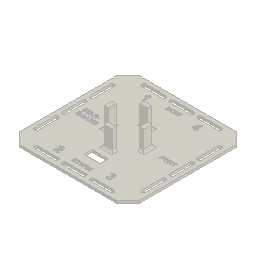
Top Plate (Autodesk Fusion 360 design; units mm, degrees)
Autodesk Fusion 360 part; units mm, degrees
sketch "Sketch1" plane through (0, 0, 0) normal (0, 0, 1) x (1, 0, 0)
  line L0 (0, 0) -> (150, 0)
  line L1 (150, 0) -> (150, 150)
  line L2 (150, 150) -> (0, 150)
  line L3 (0, 150) -> (0, 0)
  line L4 (0, 135.8579) -> (14.1421, 150)
  line L5 (0, 135.8579) -> (21.2132, 135.8579) construction
  line L6 (150, 135.8579) -> (135.8579, 150)
  line L7 (150, 135.8579) -> (176.9741, 135.8579) construction
  line L8 (0, 14.1421) -> (14.1421, 0)
  line L9 (0, 14.1421) -> (24.9877, 14.1421) construction
  line L10 (135.8579, 0) -> (150, 14.1421)
  line L11 (135.8579, 0) -> (156.2132, 0) construction
  line L12 (75, 150) -> (75, 0) construction
  line L13 (0, 75) -> (150, 75) construction
  line L14 (65, 40) -> (85, 40)
  line L15 (85, 40) -> (85, 30)
  line L16 (85, 30) -> (65, 30)
  line L17 (65, 30) -> (65, 40)
  line L18 (62, 145) -> (88, 145)
  line L19 (90, 143) -> (90, 142)
  line L20 (88, 140) -> (62, 140)
  line L21 (60, 142) -> (60, 143)
  line L22 (97, 145) -> (123, 145)
  line L23 (125, 143) -> (125, 142)
  line L24 (123, 140) -> (97, 140)
  line L25 (95, 142) -> (95, 143)
  line L26 (53, 145) -> (27, 145)
  line L27 (25, 143) -> (25, 142)
  line L28 (27, 140) -> (53, 140)
  line L29 (55, 142) -> (55, 143)
  arc A0 (27, 145) -> (25, 143) centre (27, 143) ccw
  arc A1 (25, 142) -> (27, 140) centre (27, 142) ccw
  arc A2 (53, 140) -> (55, 142) centre (53, 142) ccw
  arc A3 (55, 143) -> (53, 145) centre (53, 143) ccw
  arc A4 (62, 145) -> (60, 143) centre (62, 143) ccw
  arc A5 (60, 142) -> (62, 140) centre (62, 142) ccw
  arc A6 (90, 143) -> (88, 145) centre (88, 143) ccw
  arc A7 (88, 140) -> (90, 142) centre (88, 142) ccw
  arc A8 (95, 142) -> (97, 140) centre (97, 142) ccw
  arc A9 (97, 145) -> (95, 143) centre (97, 143) ccw
  arc A10 (125, 143) -> (123, 145) centre (123, 143) ccw
  arc A11 (123, 140) -> (125, 142) centre (123, 142) ccw
  line L30 (5, 53) -> (5, 27)
  line L31 (5, 97) -> (5, 123)
  arc A12 (10, 88) -> (8, 90) centre (8, 88) ccw
  arc A13 (8, 60) -> (10, 62) centre (8, 62) ccw
  line L32 (10, 88) -> (10, 62)
  line L33 (7, 25) -> (8, 25)
  line L34 (10, 123) -> (10, 97)
  line L35 (10, 27) -> (10, 53)
  line L36 (8, 60) -> (7, 60)
  line L37 (5, 62) -> (5, 88)
  arc A14 (7, 55) -> (5, 53) centre (7, 53) ccw
  arc A15 (10, 53) -> (8, 55) centre (8, 53) ccw
  arc A16 (5, 27) -> (7, 25) centre (7, 27) ccw
  arc A17 (7, 90) -> (5, 88) centre (7, 88) ccw
  arc A18 (8, 95) -> (10, 97) centre (8, 97) ccw
  arc A19 (10, 123) -> (8, 125) centre (8, 123) ccw
  arc A20 (7, 125) -> (5, 123) centre (7, 123) ccw
  line L38 (8, 55) -> (7, 55)
  arc A21 (5, 97) -> (7, 95) centre (7, 97) ccw
  arc A22 (5, 62) -> (7, 60) centre (7, 62) ccw
  line L39 (7, 90) -> (8, 90)
  line L40 (8, 95) -> (7, 95)
  line L41 (7, 125) -> (8, 125)
  arc A23 (8, 25) -> (10, 27) centre (8, 27) ccw
  line L42 (97, 5) -> (123, 5)
  line L43 (53, 5) -> (27, 5)
  arc A24 (62, 10) -> (60, 8) centre (62, 8) ccw
  arc A25 (90, 8) -> (88, 10) centre (88, 8) ccw
  line L44 (62, 10) -> (88, 10)
  line L45 (125, 7) -> (125, 8)
  line L46 (27, 10) -> (53, 10)
  line L47 (123, 10) -> (97, 10)
  line L48 (90, 8) -> (90, 7)
  line L49 (88, 5) -> (62, 5)
  arc A26 (95, 7) -> (97, 5) centre (97, 7) ccw
  arc A27 (97, 10) -> (95, 8) centre (97, 8) ccw
  arc A28 (123, 5) -> (125, 7) centre (123, 7) ccw
  arc A29 (60, 7) -> (62, 5) centre (62, 7) ccw
  arc A30 (55, 8) -> (53, 10) centre (53, 8) ccw
  arc A31 (27, 10) -> (25, 8) centre (27, 8) ccw
  arc A32 (25, 7) -> (27, 5) centre (27, 7) ccw
  line L50 (95, 8) -> (95, 7)
  arc A33 (53, 5) -> (55, 7) centre (53, 7) ccw
  arc A34 (88, 5) -> (90, 7) centre (88, 7) ccw
  line L51 (60, 7) -> (60, 8)
  line L52 (55, 8) -> (55, 7)
  line L53 (25, 7) -> (25, 8)
  arc A35 (125, 8) -> (123, 10) centre (123, 8) ccw
  line L54 (145, 97) -> (145, 123)
  line L55 (145, 53) -> (145, 27)
  arc A36 (140, 62) -> (142, 60) centre (142, 62) ccw
  arc A37 (142, 90) -> (140, 88) centre (142, 88) ccw
  line L56 (140, 62) -> (140, 88)
  line L57 (143, 125) -> (142, 125)
  line L58 (140, 27) -> (140, 53)
  line L59 (140, 123) -> (140, 97)
  line L60 (142, 90) -> (143, 90)
  line L61 (145, 88) -> (145, 62)
  arc A38 (143, 95) -> (145, 97) centre (143, 97) ccw
  arc A39 (140, 97) -> (142, 95) centre (142, 97) ccw
  arc A40 (145, 123) -> (143, 125) centre (143, 123) ccw
  arc A41 (143, 60) -> (145, 62) centre (143, 62) ccw
  arc A42 (142, 55) -> (140, 53) centre (142, 53) ccw
  arc A43 (140, 27) -> (142, 25) centre (142, 27) ccw
  arc A44 (143, 25) -> (145, 27) centre (143, 27) ccw
  line L62 (142, 95) -> (143, 95)
  arc A45 (145, 53) -> (143, 55) centre (143, 53) ccw
  arc A46 (145, 88) -> (143, 90) centre (143, 88) ccw
  line L63 (143, 60) -> (142, 60)
  line L64 (142, 55) -> (143, 55)
  line L65 (143, 25) -> (142, 25)
  arc A47 (142, 125) -> (140, 123) centre (142, 123) ccw
  point P0 (60, 145)
  point P1 (90, 145)
  point P2 (125, 145)
  point P3 (125, 140)
  point P4 (75, 75)
  point P5 (5, 125)
  point P6 (5, 90)
  point P7 (10, 125)
  point P8 (5, 60)
  point P9 (25, 5)
  point P10 (60, 5)
  point P11 (25, 10)
  point P12 (90, 5)
  point P13 (145, 25)
  point P14 (145, 60)
  point P15 (140, 25)
  point P16 (145, 90)
  point P17 (75, 145)
  dimension "d5" = 150
  dimension "d6" = 150
  dimension "d7" = 45
  dimension "d8" = 135
  dimension "d9" = 45
  dimension "d10" = 45
  dimension "d11" = 20
  dimension "d14" = 20
  dimension "d15" = 10
  dimension "d16" = 10
  dimension "d17" = 30
  dimension "d18" = 30
  dimension "d21" = 5
  dimension "d22" = 5
  dimension "d23" = 2
  dimension "d24" = 5
  dimension "d25" = 5
  dimension "d27" = 360
  constraint horizontal L0
  constraint vertical L1
  constraint horizontal L2
  constraint vertical L3
  constraint coincident L0.start L3.end
  constraint horizontal L5
  constraint coincident L3 L4.start
  constraint coincident L2 L4.end
  constraint horizontal L7
  constraint coincident L1 L6.start
  constraint coincident L2 L6.end
  constraint horizontal L9
  constraint coincident L3 L8.start
  constraint coincident L0 L8.end
  constraint horizontal L11
  constraint coincident L0 L10.start
  constraint coincident L1 L10.end
  constraint equal L4 L6
  constraint equal L6 L10
  constraint equal L8 L10
  constraint midpoint L2 L12.start
  constraint midpoint L0 L12.end
  constraint midpoint L3 L13.start
  constraint midpoint L1 L13.end
  constraint horizontal L14
  constraint vertical L15
  constraint horizontal L16
  constraint vertical L17
  constraint horizontal L18
  constraint vertical L19
  constraint horizontal L20
  constraint vertical L21
  constraint horizontal L22
  constraint vertical L23
  constraint horizontal L24
  constraint vertical L25
  constraint horizontal L26
  constraint vertical L27
  constraint horizontal L28
  constraint vertical L29
  constraint collinear L18 L26
  constraint collinear L18 L22
  constraint collinear L20 L28
  constraint collinear L20 L24
  constraint tangent L26 A0
  constraint tangent L27 A0
  constraint tangent L27 A1
  constraint tangent L28 A1
  constraint equal A0 A1
  constraint tangent L28 A2
  constraint tangent L29 A2
  constraint equal A0 A2
  constraint tangent L26 A3
  constraint tangent L29 A3
  constraint equal A0 A3
  constraint coincident P0 L18
  constraint coincident P0 L21
  constraint tangent L18 A4
  constraint tangent L21 A4
  constraint equal A0 A4
  constraint tangent L20 A5
  constraint tangent L21 A5
  constraint equal A0 A5
  constraint coincident P1 L18
  constraint coincident P1 L19
  constraint tangent L18 A6
  constraint tangent L19 A6
  constraint equal A0 A6
  constraint tangent L19 A7
  constraint tangent L20 A7
  constraint equal A0 A7
  constraint tangent L24 A8
  constraint tangent L25 A8
  constraint equal A0 A8
  constraint tangent L22 A9
  constraint tangent L25 A9
  constraint equal A0 A9
  constraint coincident P2 L22
  constraint coincident P2 L23
  constraint tangent L22 A10
  constraint tangent L23 A10
  constraint equal A0 A10
  constraint coincident P3 L23
  constraint coincident P3 L24
  constraint tangent L23 A11
  constraint tangent L24 A11
  constraint equal A0 A11
  constraint midpoint L13 P4
  constraint midpoint L18 P17
  constraint coincident L12 P17
  constraint equal L18 L22
  constraint equal L18 L26
  measures "d5" distance of L0.start L0.end
  measures "d6" distance of L0.start L2.end
  measures "d7" angle of L4 L5
  measures "d8" angle of L6 L7
  measures "d9" angle of L8 L9
  measures "d10" angle of L10 L11
  measures "d11" distance of L10.start L10.end
  measures "d14" distance of L15.end L16.end
  measures "d15" distance of L12 L17
  measures "d16" distance of L14.start L16.end
  measures "d17" distance of L0 L16
  measures "d18" distance of P0 P1
  measures "d21" distance of L2 L22
  measures "d22" distance of P2 P3
  measures "d23" radius of A0
  measures "d24" distance of L21 L29
  measures "d25" distance of L19 L25
extrude "Extrude1" add sketch "Sketch1" along normal blind 3 contours L0 L1 L2 L3 L4 L6 L8 L10
sketch "Sketch2" plane through (0, 0, 3) normal (0, 0, 1) x (-1, 0, 0)
  arc A0 (-5, -62) -> (-7, -60) centre (-7, -62) ccw
  line L0 (-5, -62) -> (-5, -88)
  arc A1 (-7, -90) -> (-5, -88) centre (-7, -88) ccw
  line L1 (-7, -90) -> (-8, -90)
  arc A2 (-10, -88) -> (-8, -90) centre (-8, -88) ccw
  line L2 (-10, -88) -> (-10, -62)
  arc A3 (-8, -60) -> (-10, -62) centre (-8, -62) ccw
  line L3 (-8, -60) -> (-7, -60)
  arc A4 (-142, -125) -> (-140, -123) centre (-142, -123) ccw
  line L4 (-142, -125) -> (-143, -125)
  arc A5 (-145, -123) -> (-143, -125) centre (-143, -123) ccw
  line L5 (-145, -123) -> (-145, -97)
  arc A6 (-143, -95) -> (-145, -97) centre (-143, -97) ccw
  line L6 (-143, -95) -> (-142, -95)
  arc A7 (-140, -97) -> (-142, -95) centre (-142, -97) ccw
  line L7 (-140, -97) -> (-140, -123)
  arc A8 (-88, -5) -> (-90, -7) centre (-88, -7) ccw
  line L8 (-88, -5) -> (-62, -5)
  arc A9 (-60, -7) -> (-62, -5) centre (-62, -7) ccw
  line L9 (-60, -7) -> (-60, -8)
  arc A10 (-62, -10) -> (-60, -8) centre (-62, -8) ccw
  line L10 (-62, -10) -> (-88, -10)
  arc A11 (-90, -8) -> (-88, -10) centre (-88, -8) ccw
  line L11 (-90, -8) -> (-90, -7)
  arc A12 (-145, -53) -> (-143, -55) centre (-143, -53) ccw
  line L12 (-145, -53) -> (-145, -27)
  arc A13 (-143, -25) -> (-145, -27) centre (-143, -27) ccw
  line L13 (-143, -25) -> (-142, -25)
  arc A14 (-140, -27) -> (-142, -25) centre (-142, -27) ccw
  line L14 (-140, -27) -> (-140, -53)
  arc A15 (-142, -55) -> (-140, -53) centre (-142, -53) ccw
  line L15 (-142, -55) -> (-143, -55)
  arc A16 (-125, -8) -> (-123, -10) centre (-123, -8) ccw
  line L16 (-125, -8) -> (-125, -7)
  arc A17 (-123, -5) -> (-125, -7) centre (-123, -7) ccw
  line L17 (-123, -5) -> (-97, -5)
  arc A18 (-95, -7) -> (-97, -5) centre (-97, -7) ccw
  line L18 (-95, -7) -> (-95, -8)
  arc A19 (-97, -10) -> (-95, -8) centre (-97, -8) ccw
  line L19 (-97, -10) -> (-123, -10)
  arc A20 (-53, -5) -> (-55, -7) centre (-53, -7) ccw
  line L20 (-53, -5) -> (-27, -5)
  arc A21 (-25, -7) -> (-27, -5) centre (-27, -7) ccw
  line L21 (-25, -7) -> (-25, -8)
  arc A22 (-27, -10) -> (-25, -8) centre (-27, -8) ccw
  line L22 (-27, -10) -> (-53, -10)
  arc A23 (-55, -8) -> (-53, -10) centre (-53, -8) ccw
  line L23 (-55, -8) -> (-55, -7)
  arc A24 (-145, -88) -> (-143, -90) centre (-143, -88) ccw
  line L24 (-145, -88) -> (-145, -62)
  arc A25 (-143, -60) -> (-145, -62) centre (-143, -62) ccw
  line L25 (-143, -60) -> (-142, -60)
  arc A26 (-140, -62) -> (-142, -60) centre (-142, -62) ccw
  line L26 (-140, -62) -> (-140, -88)
  arc A27 (-142, -90) -> (-140, -88) centre (-142, -88) ccw
  line L27 (-142, -90) -> (-143, -90)
  arc A28 (-5, -97) -> (-7, -95) centre (-7, -97) ccw
  line L28 (-5, -97) -> (-5, -123)
  arc A29 (-7, -125) -> (-5, -123) centre (-7, -123) ccw
  line L29 (-7, -125) -> (-8, -125)
  arc A30 (-10, -123) -> (-8, -125) centre (-8, -123) ccw
  line L30 (-10, -123) -> (-10, -97)
  arc A31 (-8, -95) -> (-10, -97) centre (-8, -97) ccw
  line L31 (-8, -95) -> (-7, -95)
  arc A32 (-95, -142) -> (-97, -140) centre (-97, -142) ccw
  line L32 (-95, -142) -> (-95, -143)
  arc A33 (-97, -145) -> (-95, -143) centre (-97, -143) ccw
  line L33 (-97, -145) -> (-123, -145)
  arc A34 (-125, -143) -> (-123, -145) centre (-123, -143) ccw
  line L34 (-125, -143) -> (-125, -142)
  arc A35 (-123, -140) -> (-125, -142) centre (-123, -142) ccw
  line L35 (-123, -140) -> (-97, -140)
  arc A36 (-60, -142) -> (-62, -140) centre (-62, -142) ccw
  line L36 (-60, -142) -> (-60, -143)
  arc A37 (-62, -145) -> (-60, -143) centre (-62, -143) ccw
  line L37 (-62, -145) -> (-88, -145)
  arc A38 (-90, -143) -> (-88, -145) centre (-88, -143) ccw
  line L38 (-90, -143) -> (-90, -142)
  arc A39 (-88, -140) -> (-90, -142) centre (-88, -142) ccw
  line L39 (-88, -140) -> (-62, -140)
  arc A40 (-55, -143) -> (-53, -145) centre (-53, -143) ccw
  line L40 (-55, -143) -> (-55, -142)
  arc A41 (-53, -140) -> (-55, -142) centre (-53, -142) ccw
  line L41 (-53, -140) -> (-27, -140)
  arc A42 (-25, -142) -> (-27, -140) centre (-27, -142) ccw
  line L42 (-25, -142) -> (-25, -143)
  arc A43 (-27, -145) -> (-25, -143) centre (-27, -143) ccw
  line L43 (-27, -145) -> (-53, -145)
  arc A44 (-8, -25) -> (-10, -27) centre (-8, -27) ccw
  line L44 (-8, -25) -> (-7, -25)
  arc A45 (-5, -27) -> (-7, -25) centre (-7, -27) ccw
  line L45 (-5, -27) -> (-5, -53)
  arc A46 (-7, -55) -> (-5, -53) centre (-7, -53) ccw
  line L46 (-7, -55) -> (-8, -55)
  arc A47 (-10, -53) -> (-8, -55) centre (-8, -53) ccw
  line L47 (-10, -53) -> (-10, -27)
  line L48 (-85, -30) -> (-65, -30)
  line L49 (-65, -30) -> (-65, -40)
  line L50 (-65, -40) -> (-85, -40)
  line L51 (-85, -40) -> (-85, -30)
  line L52 (0, -135.8579) -> (0, -14.1421)
  line L53 (0, -14.1421) -> (-14.1421, 0)
  line L54 (-14.1421, 0) -> (-135.8579, 0)
  line L55 (-135.8579, 0) -> (-150, -14.1421)
  line L56 (-150, -14.1421) -> (-150, -135.8579)
  line L57 (-150, -135.8579) -> (-135.8579, -150)
  line L58 (-135.8579, -150) -> (-14.1421, -150)
  line L59 (-14.1421, -150) -> (0, -135.8579)
  line L60 (0, 0) -> (-150, 0) construction
  line L61 (-150, 0) -> (-150, -150) construction
  line L62 (-150, -150) -> (0, -150) construction
  line L63 (0, -150) -> (0, 0) construction
  line L64 (0, -75) -> (-150, -75) construction
  line L65 (-75, -150) -> (-75, 0) construction
  line L66 (-70, -100) -> (-80, -100)
  line L67 (-80, -100) -> (-80, -95)
  line L68 (-80, -95) -> (-70, -95)
  line L69 (-70, -95) -> (-70, -100)
  line L70 (-55, -70) -> (-50, -70)
  line L71 (-55, -80) -> (-55, -70)
  line L72 (-50, -70) -> (-50, -80)
  line L73 (-50, -80) -> (-55, -80)
  line L74 (-80, -55) -> (-80, -50)
  line L75 (-70, -55) -> (-80, -55)
  line L76 (-80, -50) -> (-70, -50)
  line L77 (-70, -50) -> (-70, -55)
  line L78 (-95, -80) -> (-100, -80)
  line L79 (-95, -70) -> (-95, -80)
  line L80 (-100, -80) -> (-100, -70)
  line L81 (-100, -70) -> (-95, -70)
  point P0 (-75, -75)
  dimension "d28" = 10
  dimension "d29" = 5
  dimension "d30" = 5
  dimension "d31" = 20
  dimension "d33" = 360
  constraint horizontal L60
  constraint vertical L61
  constraint horizontal L62
  constraint vertical L63
  constraint coincident L60.start L63.end
  constraint midpoint L63 L64.start
  constraint midpoint L61 L64.end
  constraint midpoint L62 L65.start
  constraint midpoint L60 L65.end
  constraint horizontal L66
  constraint vertical L67
  constraint horizontal L68
  constraint vertical L69
  constraint midpoint L65 P0
  measures "d28" distance of L66.start L66.end
  measures "d29" distance of L65 L69
  measures "d30" distance of L66.end L67.end
  measures "d31" distance of L64 L68
extrude "Extrude2" add sketch "Sketch2" along normal blind 25 contours L66 L67 L68 L69 | L70 L71 L72 L73 | L74 L75 L76 L77 | L78 L79 L80 L81
fillet "Fillet1" radius 3 12 edges at (75, 50, 3) (80, 52.5, 3) (97.5, 70, 3) (100, 75, 3) (52.5, 70, 3) (70, 52.5, 3) (50, 75, 3) (70, 97.5, 3) (97.5, 80, 3) (75, 100, 3) (52.5, 80, 3) (80, 97.5, 3)
sketch "Sketch3" plane through (0, 0, 3) normal (0, 0, 1) x (-1, 0, 0)
  line L0 (-67, -55) -> (-83, -55)
  line L1 (-83, -55) -> (-83, -47)
  line L2 (-83, -47) -> (-67, -47)
  line L3 (-67, -47) -> (-67, -55)
  line L4 (-83, -95) -> (-67, -95)
  line L5 (-67, -95) -> (-67, -103)
  line L6 (-67, -103) -> (-83, -103)
  line L7 (-83, -103) -> (-83, -95)
  line L8 (-95, -67) -> (-95, -83)
  line L9 (-95, -83) -> (-103, -83)
  line L10 (-103, -83) -> (-103, -67)
  line L11 (-103, -67) -> (-95, -67)
  arc A0 (-5, -62) -> (-7, -60) centre (-7, -62) ccw
  line L12 (-5, -62) -> (-5, -88)
  arc A1 (-7, -90) -> (-5, -88) centre (-7, -88) ccw
  line L13 (-7, -90) -> (-8, -90)
  arc A2 (-10, -88) -> (-8, -90) centre (-8, -88) ccw
  line L14 (-10, -88) -> (-10, -62)
  arc A3 (-8, -60) -> (-10, -62) centre (-8, -62) ccw
  line L15 (-8, -60) -> (-7, -60)
  arc A4 (-142, -125) -> (-140, -123) centre (-142, -123) ccw
  line L16 (-142, -125) -> (-143, -125)
  arc A5 (-145, -123) -> (-143, -125) centre (-143, -123) ccw
  line L17 (-145, -123) -> (-145, -97)
  arc A6 (-143, -95) -> (-145, -97) centre (-143, -97) ccw
  line L18 (-143, -95) -> (-142, -95)
  arc A7 (-140, -97) -> (-142, -95) centre (-142, -97) ccw
  line L19 (-140, -97) -> (-140, -123)
  arc A8 (-88, -5) -> (-90, -7) centre (-88, -7) ccw
  line L20 (-88, -5) -> (-62, -5)
  arc A9 (-60, -7) -> (-62, -5) centre (-62, -7) ccw
  line L21 (-60, -7) -> (-60, -8)
  arc A10 (-62, -10) -> (-60, -8) centre (-62, -8) ccw
  line L22 (-62, -10) -> (-88, -10)
  arc A11 (-90, -8) -> (-88, -10) centre (-88, -8) ccw
  line L23 (-90, -8) -> (-90, -7)
  arc A12 (-145, -53) -> (-143, -55) centre (-143, -53) ccw
  line L24 (-145, -53) -> (-145, -27)
  arc A13 (-143, -25) -> (-145, -27) centre (-143, -27) ccw
  line L25 (-143, -25) -> (-142, -25)
  arc A14 (-140, -27) -> (-142, -25) centre (-142, -27) ccw
  line L26 (-140, -27) -> (-140, -53)
  arc A15 (-142, -55) -> (-140, -53) centre (-142, -53) ccw
  line L27 (-142, -55) -> (-143, -55)
  arc A16 (-125, -8) -> (-123, -10) centre (-123, -8) ccw
  line L28 (-125, -8) -> (-125, -7)
  arc A17 (-123, -5) -> (-125, -7) centre (-123, -7) ccw
  line L29 (-123, -5) -> (-97, -5)
  arc A18 (-95, -7) -> (-97, -5) centre (-97, -7) ccw
  line L30 (-95, -7) -> (-95, -8)
  arc A19 (-97, -10) -> (-95, -8) centre (-97, -8) ccw
  line L31 (-97, -10) -> (-123, -10)
  arc A20 (-53, -5) -> (-55, -7) centre (-53, -7) ccw
  line L32 (-53, -5) -> (-27, -5)
  arc A21 (-25, -7) -> (-27, -5) centre (-27, -7) ccw
  line L33 (-25, -7) -> (-25, -8)
  arc A22 (-27, -10) -> (-25, -8) centre (-27, -8) ccw
  line L34 (-27, -10) -> (-53, -10)
  arc A23 (-55, -8) -> (-53, -10) centre (-53, -8) ccw
  line L35 (-55, -8) -> (-55, -7)
  arc A24 (-145, -88) -> (-143, -90) centre (-143, -88) ccw
  line L36 (-145, -88) -> (-145, -62)
  arc A25 (-143, -60) -> (-145, -62) centre (-143, -62) ccw
  line L37 (-143, -60) -> (-142, -60)
  arc A26 (-140, -62) -> (-142, -60) centre (-142, -62) ccw
  line L38 (-140, -62) -> (-140, -88)
  arc A27 (-142, -90) -> (-140, -88) centre (-142, -88) ccw
  line L39 (-142, -90) -> (-143, -90)
  arc A28 (-5, -97) -> (-7, -95) centre (-7, -97) ccw
  line L40 (-5, -97) -> (-5, -123)
  arc A29 (-7, -125) -> (-5, -123) centre (-7, -123) ccw
  line L41 (-7, -125) -> (-8, -125)
  arc A30 (-10, -123) -> (-8, -125) centre (-8, -123) ccw
  line L42 (-10, -123) -> (-10, -97)
  arc A31 (-8, -95) -> (-10, -97) centre (-8, -97) ccw
  line L43 (-8, -95) -> (-7, -95)
  arc A32 (-95, -142) -> (-97, -140) centre (-97, -142) ccw
  line L44 (-95, -142) -> (-95, -143)
  arc A33 (-97, -145) -> (-95, -143) centre (-97, -143) ccw
  line L45 (-97, -145) -> (-123, -145)
  arc A34 (-125, -143) -> (-123, -145) centre (-123, -143) ccw
  line L46 (-125, -143) -> (-125, -142)
  arc A35 (-123, -140) -> (-125, -142) centre (-123, -142) ccw
  line L47 (-123, -140) -> (-97, -140)
  arc A36 (-60, -142) -> (-62, -140) centre (-62, -142) ccw
  line L48 (-60, -142) -> (-60, -143)
  arc A37 (-62, -145) -> (-60, -143) centre (-62, -143) ccw
  line L49 (-62, -145) -> (-88, -145)
  arc A38 (-90, -143) -> (-88, -145) centre (-88, -143) ccw
  line L50 (-90, -143) -> (-90, -142)
  arc A39 (-88, -140) -> (-90, -142) centre (-88, -142) ccw
  line L51 (-88, -140) -> (-62, -140)
  arc A40 (-55, -143) -> (-53, -145) centre (-53, -143) ccw
  line L52 (-55, -143) -> (-55, -142)
  arc A41 (-53, -140) -> (-55, -142) centre (-53, -142) ccw
  line L53 (-53, -140) -> (-27, -140)
  arc A42 (-25, -142) -> (-27, -140) centre (-27, -142) ccw
  line L54 (-25, -142) -> (-25, -143)
  arc A43 (-27, -145) -> (-25, -143) centre (-27, -143) ccw
  line L55 (-27, -145) -> (-53, -145)
  arc A44 (-8, -25) -> (-10, -27) centre (-8, -27) ccw
  line L56 (-8, -25) -> (-7, -25)
  arc A45 (-5, -27) -> (-7, -25) centre (-7, -27) ccw
  line L57 (-5, -27) -> (-5, -53)
  arc A46 (-7, -55) -> (-5, -53) centre (-7, -53) ccw
  line L58 (-7, -55) -> (-8, -55)
  arc A47 (-10, -53) -> (-8, -55) centre (-8, -53) ccw
  line L59 (-10, -53) -> (-10, -27)
  line L60 (-85, -30) -> (-65, -30)
  line L61 (-65, -30) -> (-65, -40)
  line L62 (-65, -40) -> (-85, -40)
  line L63 (-85, -40) -> (-85, -30)
  line L64 (0, -135.8579) -> (0, -14.1421)
  line L65 (0, -14.1421) -> (-14.1421, 0)
  line L66 (-14.1421, 0) -> (-135.8579, 0)
  line L67 (-135.8579, 0) -> (-150, -14.1421)
  line L68 (-150, -14.1421) -> (-150, -135.8579)
  line L69 (-150, -135.8579) -> (-135.8579, -150)
  line L70 (-135.8579, -150) -> (-14.1421, -150)
  line L71 (-14.1421, -150) -> (0, -135.8579)
  line L72 (-55, -83) -> (-55, -67)
  line L73 (-55, -67) -> (-47, -67)
  line L74 (-47, -67) -> (-47, -83)
  line L75 (-47, -83) -> (-55, -83)
  line L76 (-63.9286, -127.3047) -> (-86.0714, -127.3047) construction
  line L77 (-86.0714, -127.3047) -> (-86.0714, -135) construction
  line L78 (-86.0714, -135) -> (-63.9286, -135) construction
  line L79 (-63.9286, -135) -> (-63.9286, -127.3047) construction
  line L80 (-116, -71.5) -> (-135, -71.5) construction
  line L81 (-135, -71.5) -> (-135, -78.5) construction
  line L82 (-135, -78.5) -> (-116, -78.5) construction
  line L83 (-116, -78.5) -> (-116, -71.5) construction
  line L84 (-15, -70.5) -> (-34, -70.5) construction
  line L85 (-34, -70.5) -> (-34, -79.5) construction
  line L86 (-34, -79.5) -> (-15, -79.5) construction
  line L87 (-15, -79.5) -> (-15, -70.5) construction
  line L88 (-63.5, -15) -> (-86.5, -15) construction
  line L89 (-86.5, -15) -> (-86.5, -23) construction
  line L90 (-86.5, -23) -> (-63.5, -23) construction
  line L91 (-63.5, -23) -> (-63.5, -15) construction
  line L92 (-40, -125) -> (-45, -125) construction
  line L93 (-45, -125) -> (-45, -135) construction
  line L94 (-45, -135) -> (-40, -135) construction
  line L95 (-40, -135) -> (-40, -125) construction
  line L96 (-40, -15) -> (-48, -15) construction
  line L97 (-48, -15) -> (-48, -26) construction
  line L98 (-48, -26) -> (-40, -26) construction
  line L99 (-40, -26) -> (-40, -15) construction
  line L100 (0, -75) -> (-150, -75) construction
  line L101 (-75, 0) -> (-75, -150) construction
  line L102 (-102, -124) -> (-110, -124) construction
  line L103 (-110, -124) -> (-110, -135) construction
  line L104 (-110, -135) -> (-102, -135) construction
  line L105 (-102, -135) -> (-102, -124) construction
  line L106 (-104, -15) -> (-110, -15) construction
  line L107 (-110, -15) -> (-110, -24) construction
  line L108 (-110, -24) -> (-104, -24) construction
  line L109 (-104, -24) -> (-104, -15) construction
  dimension "d38" = 5
  dimension "d39" = 5
  dimension "d40" = 5
  dimension "d41" = 5
  dimension "d43" = 10
  dimension "d45" = 10
  dimension "d47" = 5
  dimension "d48" = 5
  dimension "d49" = 5
  dimension "d50" = 5
  dimension "d51" = 35
  dimension "d55" = 10
  dimension "d56" = 10
  dimension "d57" = 35
  text T0 "BOW" font "Arial" height 5 bold align centre top in box 22.1429 x 7.6953 at (-63.9286, -127.3047) x (-1, 0) y (0, -1) spacing 1 kerned
  text T1 "PORT" font "Arial" height 5 bold align right middle in box 19 x 7 at (-116, -71.5) x (-1, 0) y (0, -1) spacing 1 kerned
  text T2 "STAR-\nBOARD" font "Arial" height 5 bold align left middle in box 19 x 9 at (-15, -70.5) x (-1, 0) y (0, -1) spacing 1 kerned
  text T3 "STERN" font "Arial" height 5 bold align centre bottom in box 23 x 8 at (-63.5, -15) x (-1, 0) y (0, -1) spacing 1 kerned
  text T4 "1" font "Arial" height 10 bold align left top in box 5 x 10 at (-40, -125) x (-1, 0) y (0, -1) spacing 1 kerned
  text T5 "2" font "Arial" height 10 bold align left bottom in box 8 x 11 at (-40, -15) x (-1, 0) y (0, -1) spacing 1 kerned
  text T6 "4" font "Arial" height 10 bold align right top in box 8 x 11 at (-102, -124) x (-1, 0) y (0, -1) spacing 1 kerned
  text T7 "3" font "Arial" height 10 bold align right bottom in box 6 x 9 at (-104, -15) x (-1, 0) y (0, -1) spacing 1 kerned
  constraint midpoint L64 L100.start
  constraint midpoint L68 L100.end
  constraint midpoint L66 L101.start
  constraint midpoint L70 L101.end
  constraint coincident L101
  constraint coincident L100
  constraint collinear L78 L94
  constraint collinear L88 L96
  constraint collinear L95 L99
  constraint collinear L78 L104
  constraint collinear L88 L106
  constraint collinear L103 L107
  measures "d47" distance of L51 L78
  measures "d48" distance of L38 L81
  measures "d49" distance of L22 L88
  measures "d50" distance of L14 L87
  measures "d51" distance of L95 L101
  measures "d57" distance of L101 L103
extrude "Extrude3" cut sketch "Sketch3" against normal blind 1 text T0 T4 T2 T5 T3 T1 T6 T7
equation "d6 = d5"
equation "d15 = d14 / 2"
equation "d25 = d24"
equation "d29 = d28 / 2"
equation "d57 = d51"
